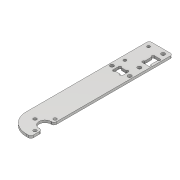
# Autodesk Inventor part: Part1
Saved by Autodesk Inventor 2017.3 (Build 213256000, 256)
## iProperties
Part Number: Part1
Material: アルミニウム 2014-T4
Document SubType Name: Modeling
Designer: haya
Density: 2.8 g/cm^3
Appearance: サテン
Author: haya
Autodesk Inventor part; units mm, degrees
ref_plane "YZ Plane" through (0, 0, 0) normal (1, 0, 0) x (0, 1, 0)
ref_plane "XZ Plane" through (0, 0, 0) normal (0, 1, 0) x (-1, 0, 0)
ref_plane "XY Plane" through (0, 0, 0) normal (0, 0, 1) x (1, 0, 0)
sketch "スケッチ1" plane through (0, 0, 0) normal (0, 0, 1) x (1, 0, 0)
  line L0 (0, 0) -> (20, 0)
  line L1 (20, 0) -> (20, 120)
  line L2 (20, 120) -> (0, 120)
  line L3 (0, 120) -> (0, 0)
  dimension "d0" = 120
  dimension "d1" = 20
  constraints: 8 end point, 2 parallel, 1 horizontal, 1 perpendicular
  measures "d0" distance of L2.end L0.start
  measures "d1" distance of L0.start L0.end
extrude "押し出し1" add sketch "スケッチ1" along normal blind 2
sketch "スケッチ2" plane through (0, 0, 2) normal (0, 0, 1) x (1, 0, 0)
  line L0 (0, 0) -> (20, 0) projected
  line L1 (17.5, 0) -> (17.5, 120.1891) construction
  line L2 (20, 0) -> (20, 120) projected
  arc A0 (17.5, 19.55) -> (17.5, 9.45) centre (17.5, 14.5) ccw
  line L3 (17.5, 19.55) -> (20, 19.55)
  line L4 (17.5, 9.45) -> (20, 9.45)
  dimension "d4" = 2.5
  dimension "d5" = 14.5
  dimension "d6" = 10.1
  constraints: 6 end point, 6 point on line, 2 perpendicular, 2 point on circle, 2 tangent, 1 centre point, 1 coincident, 1 vertical
  measures "d4" distance between parallel lines of L1 L2
  measures "d5" distance from line of point (17.5, 14.5) L0
  measures "d6" diameter of A0
extrude "押し出し2" cut sketch "スケッチ2" against normal up to surface (2 mm away)
sketch "スケッチ3" plane through (0, 0, 2) normal (0, 0, 1) x (1, 0, 0)
  arc A0 (17.5, 19.55) -> (17.5, 9.45) centre (17.5, 14.5) ccw projected
  circle A1 centre (17.5, 14.5) radius 8.5 construction
  point P0 (0, 0)
  point P1 (9, 14.5)
  point P2 (17.5, 23)
  point P3 (17.5, 6)
  dimension "d9" = 17
  constraints: 3 point on circle, 1 centre point, 1 coincident
  measures "d9" diameter of A1
hole "穴1" at (9, 14.5, 2) at (17.5, 23, 2) at (17.5, 6, 2) direction (0, 0, -1) diameter 2.7 end through all
sketch "スケッチ4" plane through (0, 0, 2) normal (0, 0, 1) x (1, 0, 0)
  line L0 (20, 120) -> (0, 120) projected
  line L1 (4, 120) -> (4, 0) construction
  line L2 (0, 120) -> (0, 0) projected
  point P0 (4, 115.5)
  point P1 (4, 95.5)
  dimension "d17" = 4
  dimension "d18" = 4.5
  dimension "d19" = 20
  constraints: 3 point on line, 2 end point, 1 perpendicular
  measures "d17" distance between parallel lines of L1 L2
  measures "d18" distance from line of point (4, 115.5) L0
  measures "d19" distance of point (4, 95.5) point (4, 115.5)
hole "穴2" at (4, 115.5, 2) at (4, 95.5, 2) direction (0, 0, -1) diameter 2.4 end through all
sketch "スケッチ5" plane through (0, 0, 2) normal (0, 0, 1) x (1, 0, 0)
  line L0 (13, 111.275) -> (18, 111.275)
  line L1 (18, 111.275) -> (18, 101.275)
  line L2 (18, 101.275) -> (13, 101.275)
  line L3 (13, 101.275) -> (13, 111.275)
  line L4 (20, 19.55) -> (20, 120) projected
  circle A0 centre (18, 110.275) radius 1
  circle A1 centre (13, 110.275) radius 1
  circle A2 centre (13, 102.275) radius 1
  circle A3 centre (18, 102.275) radius 1
  point P0 (0, 0)
  dimension "d27" = 5
  dimension "d28" = 10
  dimension "d29" = 2
  dimension "d30" = 2
  dimension "d31" = 2
  dimension "d32" = 2
  dimension "d33" = 2
  constraints: 8 end point, 4 centre point, 4 point on line, 4 tangent, 2 parallel, 1 horizontal, 1 perpendicular
  measures "d27" distance of L0.start L0.end
  measures "d28" distance of L0.end L1.end
  measures "d29" distance between parallel lines of L4 L1
  measures "d30" diameter of A0
  measures "d31" diameter of A1
  measures "d32" diameter of A2
  measures "d33" diameter of A3
extrude "押し出し3" cut sketch "スケッチ5" against normal up to surface (2 mm away)
sketch "スケッチ6" plane through (0, 0, 2) normal (0, 0, 1) x (1, 0, 0)
  line L0 (15.5, 119.9651) -> (15.5, 0) construction
  line L1 (0, 0) -> (20, 0) projected
  line L2 (18, 109.275) -> (18, 103.275) projected
  line L3 (18, 106.275) -> (13, 106.275) construction
  line L4 (13, 103.275) -> (13, 109.275) projected
  point P0 (15.5, 116.275)
  point P1 (15.5, 96.275)
  dimension "d37" = 2.5
  dimension "d38" = 20
  constraints: 4 end point, 2 midpoint, 2 point on line, 1 symmetric about line, 1 vertical
  measures "d37" distance between parallel lines of L0 L2
  measures "d38" distance of point (15.5, 96.275) point (15.5, 116.275)
hole "穴3" at (15.5, 116.275, 2) at (15.5, 96.275, 2) direction (0, 0, -1) diameter 3.1 end through all
sketch "スケッチ7" plane through (0, 0, 2) normal (0, 0, 1) x (1, 0, 0)
  line L0 (20, 120) -> (0, 120) projected
  line L1 (10, 120) -> (10, 0) construction
  line L2 (0, 0) -> (20, 0) projected
  line L3 (8, 88.5) -> (12, 88.5)
  line L4 (14, 88.5) -> (14, 83.5)
  line L5 (12, 83.5) -> (8, 83.5)
  line L6 (6, 83.5) -> (6, 88.5)
  arc A0 (8, 88.5) -> (6, 88.5) centre (7, 88.5) ccw
  line L7 (6, 86) -> (14, 86) construction
  arc A1 (6, 83.5) -> (8, 83.5) centre (7, 83.5) ccw
  arc A2 (14, 88.5) -> (12, 88.5) centre (13, 88.5) ccw
  arc A3 (12, 83.5) -> (14, 83.5) centre (13, 83.5) ccw
  dimension "d48" = 8
  dimension "d49" = 5
  dimension "d50" = 2
  dimension "d64" = 34
  constraints: 12 end point, 8 point on circle, 4 centre point, 4 midpoint, 3 symmetric about line, 2 parallel, 1 horizontal, 1 perpendicular, 1 point on line, 1 tangent, 4 other
  measures "d48" distance of L4.end L6.start
  measures "d49" distance of L4.start L4.end
  measures "d50" diameter of A0
  measures "d64" distance between parallel lines of L7 L0
extrude "押し出し5" cut sketch "スケッチ7" against normal through all
sketch "スケッチ9" plane through (0, 0, 2) normal (0, 0, 1) x (1, 0, 0)
  line L0 (0, 86) -> (19.9715, 86) construction
  line L1 (8, 88.5) -> (12, 88.5) projected
  line L2 (10, 88.5) -> (10, 71.9666) construction
  point P0 (0, 0)
  point P1 (2.5, 86)
  point P2 (17.5, 86)
  dimension "d55" = 2.5
  dimension "d56" = 15
  constraints: 4 end point, 1 horizontal, 1 midpoint, 1 point on line, 1 symmetric about line, 1 vertical
  measures "d55" distance between parallel lines of L0 L1
  measures "d56" distance of point (17.5, 86) point (2.5, 86)
hole "穴4" at (2.5, 86, 2) at (17.5, 86, 2) direction (0, 0, -1) diameter 3.1 end through all
fillet "フィレット3" radius 2 5 edges at (20, 0, 1) (20, 9.45, 1) (20, 19.55, 1) (20, 120, 1) (0, 120, 1)
fillet "フィレット4" radius 16 1 edges at (0, 0, 1)
thicken "厚み1" operation cut thickness 0.05 both sides no extend neighbours no toward (-1, 0, 0) faces at (6, 86.8333, 1.3333) (7.7994, 89.1007, 0.6667) (10.6667, 88.5, 0.6667) (12.1548, 89.0345, 0.6667) (6.2006, 82.8993, 0.6667) (9.3333, 83.5, 1.3333) (12.08, 83.108, 0.6667) (14, 85.1667, 1.3333)
thicken "厚み2" operation cut thickness 0.05 both sides no extend neighbours no toward (1, 0, 0) faces at (18, 107.275, 1.3333) (18.866, 110.775, 0.6667) (18.9035, 101.8464, 1.3333) (16.3333, 101.275, 1.3333) (12.0008, 102.2348, 0.6667) (13, 105.275, 1.3333) (12.134, 109.775, 0.6667) (14.6667, 111.275, 1.3333)
equation "\"d37\" = 0.5 * d27"
equation "\"d55\" = 0.5 * d49"
